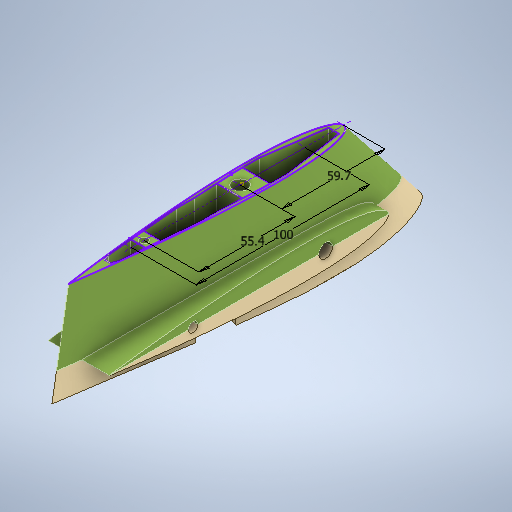
# Autodesk Inventor part: adjusted emp joint
Saved by Autodesk Inventor 2025.2 (Build 292293000, 293)
## iProperties
Created: 2025-01-22
Part Number: adjusted emp joint
Material: Generic
Document SubType Name: Modeling
Designer: User
Density: 1 g/cm^3
Appearance: Default
Author: User
Autodesk Inventor part; units mm, degrees
sketch "Sketch2" plane through (0, 0, 0) normal (0, 1, 0) x (-1, 0, 0)
  spline S0 degree 4 poles (0, 110.7513) (-0.0049, 110.7185) (-0.0278, 110.5585) (-0.067, 110.2903) (-0.1327, 109.8368) (-0.2012, 109.3601) (-0.2858, 108.7746) (-0.3847, 108.0848) (-0.4979, 107.2904) (-0.6258, 106.3921) (-0.7667, 105.3911) (-0.922, 104.2884) (-1.0895, 103.0852) (-1.2699, 101.7823) (-1.4624, 100.3817) (-1.6663, 98.8837) (-1.8812, 97.2908) (-2.107, 95.6041) (-2.3421, 93.8253) (-2.5871, 91.9562) (-2.8408, 89.9986) (-3.1031, 87.9548) (-3.3721, 85.826) (-3.6492, 83.6152) (-3.9321, 81.3238) (-4.2206, 78.9546) (-4.5149, 76.51) (-4.8135, 73.9919) (-5.116, 71.4031) (-5.4221, 68.7463) (-5.7308, 66.0238) (-6.0411, 63.2385) (-6.3537, 60.3929) (-6.6665, 57.4903) (-6.9799, 54.5331) (-7.2921, 51.5242) (-7.604, 48.4671) (-7.914, 45.3643) (-8.2212, 42.2189) (-8.5257, 39.0344) (-8.8259, 35.8132) (-9.1221, 32.5597) (-9.4131, 29.2757) (-9.6978, 25.9654) (-9.9763, 22.6318) (-10.2471, 19.2778) (-10.5104, 15.9076) (-10.7638, 12.5235) (-11.0089, 9.1296) (-11.2424, 5.7289) (-11.4659, 2.325) (-11.6768, -1.079) (-11.875, -4.4797) (-12.06, -7.8736) (-12.2312, -11.2577) (-12.3866, -14.628) (-12.5273, -17.982) (-12.651, -21.3157) (-12.7583, -24.626) (-12.8475, -27.91) (-12.9186, -31.1637) (-12.971, -34.3849) (-13.0036, -37.5695) (-13.0168, -40.7149) (-13.0094, -43.818) (-12.9816, -46.8752) (-12.9328, -49.8841) (-12.8624, -52.8415) (-12.7706, -55.7442) (-12.6573, -58.5901) (-12.5219, -61.3755) (-12.3652, -64.0983) (-12.1863, -66.7553) (-11.9859, -69.3443) (-11.7639, -71.8627) (-11.5213, -74.3077) (-11.2571, -76.6772) (-10.9725, -78.9689) (-10.6682, -81.1803) (-10.3438, -83.3094) (-10.0001, -85.3538) (-9.6381, -87.312) (-9.2577, -89.1818) (-8.8603, -90.9614) (-8.4459, -92.649) (-8.0154, -94.243) (-7.5694, -95.7422) (-7.1089, -97.1444) (-6.6339, -98.4491) (-6.1459, -99.6547) (-5.6448, -100.7602) (-5.1315, -101.7646) (-4.607, -102.6674) (-4.0703, -103.4669) (-3.5231, -104.1642) (-2.9644, -104.757) (-2.3942, -105.2456) (-1.8122, -105.6289) (-1.218, -105.9043) (-0.6135, -106.0703) (0, -106.1253) (0.6135, -106.0703) (1.218, -105.9043) (1.8122, -105.6289) (2.3942, -105.2456) (2.9644, -104.757) (3.5231, -104.1642) (4.0703, -103.4669) (4.607, -102.6674) (5.1315, -101.7646) (5.6448, -100.7602) (6.1459, -99.6547) (6.6339, -98.4491) (7.1089, -97.1444) (7.5694, -95.7422) (8.0154, -94.243) (8.4459, -92.649) (8.8603, -90.9614) (9.2577, -89.1818) (9.6381, -87.312) (10.0001, -85.3538) (10.3438, -83.3094) (10.6682, -81.1803) (10.9725, -78.9689) (11.2571, -76.6772) (11.5213, -74.3077) (11.7639, -71.8627) (11.9859, -69.3443) (12.1863, -66.7553) (12.3652, -64.0983) (12.5219, -61.3755) (12.6573, -58.5901) (12.7706, -55.7442) (12.8624, -52.8415) (12.9328, -49.8841) (12.9816, -46.8752) (13.0094, -43.818) (13.0168, -40.7149) (13.0036, -37.5695) (12.971, -34.3849) (12.9186, -31.1637) (12.8475, -27.91) (12.7583, -24.626) (12.651, -21.3157) (12.5273, -17.982) (12.3866, -14.628) (12.2312, -11.2577) (12.06, -7.8736) (11.875, -4.4797) (11.6768, -1.079) (11.4659, 2.325) (11.2424, 5.7289) (11.0089, 9.1296) (10.7638, 12.5235) (10.5104, 15.9076) (10.2471, 19.2778) (9.9763, 22.6318) (9.6978, 25.9654) (9.4131, 29.2757) (9.1221, 32.5597) (8.8259, 35.8132) (8.5257, 39.0344) (8.2212, 42.2189) (7.914, 45.3643) (7.604, 48.4671) (7.2921, 51.5242) (6.9799, 54.5331) (6.6665, 57.4903) (6.3537, 60.3929) (6.0411, 63.2385) (5.7308, 66.0238) (5.4221, 68.7463) (5.116, 71.4031) (4.8135, 73.9919) (4.5149, 76.51) (4.2206, 78.9546) (3.9321, 81.3238) (3.6492, 83.6152) (3.3721, 85.826) (3.1031, 87.9548) (2.8408, 89.9986) (2.5871, 91.9562) (2.3421, 93.8253) (2.107, 95.6041) (1.8812, 97.2908) (1.6663, 98.8837) (1.4624, 100.3817) (1.2699, 101.7823) (1.0895, 103.0852) (0.922, 104.2884) (0.7667, 105.3911) (0.6258, 106.3921) (0.4979, 107.2904) (0.3847, 108.0848) (0.2858, 108.7746) (0.2012, 109.3601) (0.1327, 109.8368) (0.067, 110.2903) (0.0278, 110.5585) (0.0049, 110.7185) (0, 110.7513) knots 0 0 0 0 0 0.003305 0.005251 0.007517 0.010057 0.012844 0.015853 0.019069 0.022477 0.026064 0.029821 0.033738 0.037807 0.04202 0.046371 0.050853 0.05546 0.060186 0.065027 0.069976 0.07503 0.080184 0.085434 0.090774 0.096201 0.101711 0.1073 0.112964 0.118699 0.124501 0.130368 0.136295 0.142278 0.148315 0.154402 0.160535 0.166711 0.172927 0.179179 0.185465 0.19178 0.198121 0.204486 0.210871 0.217273 0.223689 0.230115 0.236548 0.242985 0.249423 0.255859 0.262289 0.268711 0.275121 0.281516 0.287892 0.294248 0.300579 0.306882 0.313155 0.319394 0.325595 0.331757 0.337875 0.343946 0.349967 0.355935 0.361846 0.367698 0.373486 0.379209 0.384861 0.390441 0.395943 0.401366 0.406705 0.411957 0.417118 0.422185 0.427153 0.432019 0.436778 0.441428 0.445964 0.450381 0.454676 0.458845 0.462884 0.466789 0.470556 0.474184 0.477671 0.481017 0.484224 0.487301 0.490258 0.493116 0.495899 0.498638 0.501362 0.504101 0.506884 0.509742 0.512699 0.515776 0.518983 0.522329 0.525816 0.529444 0.533211 0.537116 0.541155 0.545324 0.549619 0.554036 0.558572 0.563222 0.567981 0.572847 0.577815 0.582882 0.588043 0.593295 0.598634 0.604057 0.609559 0.615139 0.620791 0.626514 0.632302 0.638154 0.644065 0.650033 0.656054 0.662125 0.668243 0.674405 0.680606 0.686845 0.693118 0.699421 0.705752 0.712108 0.718484 0.724879 0.731289 0.737711 0.744141 0.750577 0.757015 0.763452 0.769885 0.776311 0.782727 0.789129 0.795514 0.801879 0.80822 0.814535 0.820821 0.827073 0.833289 0.839465 0.845598 0.851685 0.857722 0.863705 0.869632 0.875499 0.881301 0.887036 0.8927 0.898289 0.903799 0.909226 0.914566 0.919816 0.92497 0.930024 0.934973 0.939814 0.94454 0.949147 0.953629 0.95798 0.962193 0.966262 0.970179 0.973936 0.977523 0.980931 0.984147 0.987156 0.989943 0.992483 0.994749 0.996695 1 1 1 1 1
  line L0 (-10.6258, 14.3547) -> (0, 14.3547)
  line L1 (0, 14.3547) -> (0, 35.8301)
  line L2 (0, 35.8301) -> (-8.8229, 35.8301)
  point P0 (0, 0)
  point P1 (0, 0)
  point P2 (0, 109.384)
  point P3 (0, -106.1025)
  point P4 (0, 0)
  point P5 (0, -106.1025)
  point P6 (-0.031, 110.5373)
  point P7 (-0.0698, 110.2701)
  point P8 (-0.124, 109.8962)
  point P9 (-0.1932, 109.4163)
  point P10 (-0.2776, 108.8308)
  point P11 (-0.3767, 108.1399)
  point P12 (-0.4901, 107.345)
  point P13 (-0.6178, 106.4461)
  point P14 (-0.7592, 105.4445)
  point P15 (-0.9143, 104.3411)
  point P16 (-1.0821, 103.1371)
  point P17 (-1.2625, 101.8336)
  point P18 (-1.4551, 100.4321)
  point P19 (-1.6591, 98.9334)
  point P20 (-1.8743, 97.3395)
  point P21 (-2.1, 95.652)
  point P22 (-2.3355, 93.8723)
  point P23 (-2.5806, 92.0021)
  point P24 (-2.8345, 90.0435)
  point P25 (-3.0967, 87.9986)
  point P26 (-3.3662, 85.8688)
  point P27 (-3.6431, 83.6567)
  point P28 (-3.9264, 81.3641)
  point P29 (-4.2152, 78.9937)
  point P30 (-4.5095, 76.5478)
  point P31 (-4.8083, 74.0284)
  point P32 (-5.111, 71.4383)
  point P33 (-5.4172, 68.7801)
  point P34 (-5.726, 66.0562)
  point P35 (-6.0368, 63.2694)
  point P36 (-6.3493, 60.4224)
  point P37 (-6.6624, 57.5183)
  point P38 (-6.9758, 54.5595)
  point P39 (-7.2885, 51.5491)
  point P40 (-7.6003, 48.4904)
  point P41 (-7.9104, 45.3859)
  point P42 (-8.2179, 42.239)
  point P43 (-8.5224, 39.0527)
  point P44 (-9.1191, 32.5746)
  point P45 (-9.4102, 29.2891)
  point P46 (-9.6951, 25.9771)
  point P47 (-9.9735, 22.6417)
  point P48 (-10.2446, 19.2861)
  point P49 (-10.5076, 15.914)
  point P50 (-10.7616, 12.5282)
  point P51 (-11.0062, 9.1325)
  point P52 (-11.2402, 5.7301)
  point P53 (-11.4633, 2.3244)
  point P54 (-11.6743, -1.0813)
  point P55 (-11.8725, -4.4837)
  point P56 (-12.0575, -7.8794)
  point P57 (-12.2284, -11.2652)
  point P58 (-12.3841, -14.6372)
  point P59 (-12.5244, -17.9928)
  point P60 (-12.6482, -21.3283)
  point P61 (-12.7551, -24.6403)
  point P62 (-12.8442, -27.9258)
  point P63 (-12.9152, -31.1812)
  point P64 (-12.9672, -34.4039)
  point P65 (-12.9997, -37.5901)
  point P66 (-13.0125, -40.7371)
  point P67 (-13.0049, -43.8416)
  point P68 (-12.9767, -46.9003)
  point P69 (-12.9275, -49.9107)
  point P70 (-12.8568, -52.8694)
  point P71 (-12.7647, -55.7735)
  point P72 (-12.6508, -58.6206)
  point P73 (-12.5151, -61.4074)
  point P74 (-12.3576, -64.1313)
  point P75 (-12.1783, -66.7895)
  point P76 (-11.9773, -69.3796)
  point P77 (-11.7548, -71.899)
  point P78 (-11.5112, -74.3449)
  point P79 (-11.2465, -76.7153)
  point P80 (-10.9611, -79.0079)
  point P81 (-10.6558, -81.22)
  point P82 (-10.3305, -83.3497)
  point P83 (-9.9859, -85.3947)
  point P84 (-9.6227, -87.3533)
  point P85 (-9.2412, -89.2234)
  point P86 (-8.8424, -91.0032)
  point P87 (-8.4267, -92.6907)
  point P88 (-7.9947, -94.2846)
  point P89 (-7.5472, -95.7833)
  point P90 (-7.0848, -97.1848)
  point P91 (-6.6082, -98.4883)
  point P92 (-6.1181, -99.6923)
  point P93 (-5.615, -100.7956)
  point P94 (-5.0998, -101.7973)
  point P95 (-4.573, -102.6961)
  point P96 (-4.035, -103.4911)
  point P97 (-3.4866, -104.182)
  point P98 (-2.9282, -104.7675)
  point P99 (-2.3602, -105.2474)
  point P100 (-1.7832, -105.6213)
  point P101 (-1.1973, -105.8884)
  point P102 (-0.6026, -106.0489)
  point P103 (0, -106.1025)
  point P104 (0.6026, -106.0489)
  point P105 (1.1973, -105.8884)
  point P106 (1.7832, -105.6213)
  point P107 (2.3602, -105.2474)
  point P108 (2.9282, -104.7675)
  point P109 (3.4866, -104.182)
  point P110 (4.035, -103.4911)
  point P111 (4.573, -102.6961)
  point P112 (5.0998, -101.7973)
  point P113 (5.615, -100.7956)
  point P114 (6.1181, -99.6923)
  point P115 (6.6082, -98.4883)
  point P116 (7.0848, -97.1848)
  point P117 (7.5472, -95.7833)
  point P118 (7.9947, -94.2846)
  point P119 (8.4267, -92.6907)
  point P120 (8.8424, -91.0032)
  point P121 (9.2412, -89.2234)
  point P122 (9.6227, -87.3533)
  point P123 (9.9859, -85.3947)
  point P124 (10.3305, -83.3497)
  point P125 (10.6558, -81.22)
  point P126 (10.9611, -79.0079)
  point P127 (11.2465, -76.7153)
  point P128 (11.5112, -74.3449)
  point P129 (11.7548, -71.899)
  point P130 (11.9773, -69.3796)
  point P131 (12.1783, -66.7895)
  point P132 (12.3576, -64.1313)
  point P133 (12.5151, -61.4074)
  point P134 (12.6508, -58.6206)
  point P135 (12.7647, -55.7735)
  point P136 (12.8568, -52.8694)
  point P137 (12.9275, -49.9107)
  point P138 (12.9767, -46.9003)
  point P139 (13.0049, -43.8416)
  point P140 (13.0125, -40.7371)
  point P141 (12.9997, -37.5901)
  point P142 (12.9672, -34.4039)
  point P143 (12.9152, -31.1812)
  point P144 (12.8442, -27.9258)
  point P145 (12.7551, -24.6403)
  point P146 (12.6482, -21.3283)
  point P147 (12.5244, -17.9928)
  point P148 (12.3841, -14.6372)
  point P149 (12.2284, -11.2652)
  point P150 (12.0575, -7.8794)
  point P151 (11.8725, -4.4837)
  point P152 (11.6743, -1.0813)
  point P153 (11.4633, 2.3244)
  point P154 (11.2402, 5.7301)
  point P155 (11.0062, 9.1325)
  point P156 (10.7616, 12.5282)
  point P157 (10.5076, 15.914)
  point P158 (10.2446, 19.2861)
  point P159 (9.9735, 22.6417)
  point P160 (9.6951, 25.9771)
  point P161 (9.4102, 29.2891)
  point P162 (9.1191, 32.5746)
  point P163 (8.8229, 35.8301)
  point P164 (8.5224, 39.0527)
  point P165 (8.2179, 42.239)
  point P166 (7.9104, 45.3859)
  point P167 (7.6003, 48.4904)
  point P168 (7.2885, 51.5491)
  point P169 (6.9758, 54.5595)
  point P170 (6.6624, 57.5183)
  point P171 (6.3493, 60.4224)
  point P172 (6.0368, 63.2694)
  point P173 (5.726, 66.0562)
  point P174 (5.4172, 68.7801)
  point P175 (5.111, 71.4383)
  point P176 (4.8083, 74.0284)
  point P177 (4.5095, 76.5478)
  point P178 (4.2152, 78.9937)
  point P179 (3.9264, 81.3641)
  point P180 (3.6431, 83.6567)
  point P181 (3.3662, 85.8688)
  point P182 (3.0967, 87.9986)
  point P183 (2.8345, 90.0435)
  point P184 (2.5806, 92.0021)
  point P185 (2.3355, 93.8723)
  point P186 (2.1, 95.652)
  point P187 (1.8743, 97.3395)
  point P188 (1.6591, 98.9334)
  point P189 (1.4551, 100.4321)
  point P190 (1.2625, 101.8336)
  point P191 (1.0821, 103.1371)
  point P192 (0.9143, 104.3411)
  point P193 (0.7592, 105.4445)
  point P194 (0.6178, 106.4461)
  point P195 (0.4901, 107.345)
  point P196 (0.3767, 108.1399)
  point P197 (0.2776, 108.8308)
  point P198 (0.1932, 109.4163)
  point P199 (0.124, 109.8962)
  constraints: 6 end point, 2 coincident, 1 horizontal, 1 parallel, 1 perpendicular, 203 other
ref_plane "Work Plane1" through (0, 60, 0) normal (0, 1, 0) x (-1, 0, 0)
sketch "Sketch3" plane through (0, 60, 0) normal (0, 1, 0) x (-1, 0, 0)
  line L0 (-3, -52.6917) -> (-8, -17.6917)
  line L1 (8, -17.6917) -> (3, -52.6917)
  line L2 (3, -52.6917) -> (-3, -52.6917)
  line L3 (-1.6981, 77.7583) -> (1.6981, 77.7583)
  line L4 (1.6981, 77.7583) -> (3, 74.3083)
  line L5 (3, 74.3083) -> (6.7391, 31.3083)
  line L6 (-6.7391, 31.3083) -> (-3, 74.3083)
  line L7 (-3, 74.3083) -> (-1.6981, 77.7583)
  spline S0 degree 4 poles (0, 100.3083) (0.0036, 100.2843) (0.0203, 100.1673) (0.049, 99.9711) (0.0971, 99.6395) (0.1472, 99.2908) (0.209, 98.8626) (0.2814, 98.358) (0.3641, 97.777) (0.4577, 97.1201) (0.5608, 96.388) (0.6743, 95.5815) (0.7968, 94.7015) (0.9287, 93.7486) (1.0695, 92.7242) (1.2187, 91.6287) (1.3758, 90.4637) (1.541, 89.2301) (1.713, 87.9291) (1.8922, 86.5621) (2.0777, 85.1304) (2.2695, 83.6356) (2.4662, 82.0787) (2.6689, 80.4618) (2.8758, 78.7859) (3.0868, 77.0532) (3.3021, 75.2653) (3.5205, 73.4236) (3.7417, 71.5303) (3.9656, 69.5872) (4.1913, 67.596) (4.4183, 65.5589) (4.6469, 63.4777) (4.8756, 61.3549) (5.1049, 59.192) (5.3332, 56.9915) (5.5613, 54.7556) (5.788, 52.4862) (6.0127, 50.1858) (6.2354, 47.8568) (6.455, 45.5009) (6.6716, 43.1214) (6.8844, 40.7196) (7.0927, 38.2986) (7.2964, 35.8604) (7.4944, 33.4075) (7.687, 30.9426) (7.8723, 28.4676) (8.0516, 25.9854) (8.2223, 23.4982) (8.3858, 21.0087) (8.54, 18.5191) (8.685, 16.0319) (8.8203, 13.5498) (8.9455, 11.0747) (9.0592, 8.6098) (9.1621, 6.1568) (9.2526, 3.7186) (9.331, 1.2976) (9.3962, -1.1042) (9.4483, -3.4839) (9.4866, -5.8398) (9.5104, -8.1689) (9.5201, -10.4694) (9.5147, -12.7388) (9.4943, -14.9748) (9.4586, -17.1754) (9.4071, -19.3384) (9.34, -21.4613) (9.2572, -23.5427) (9.1581, -25.5799) (9.0435, -27.5712) (8.9126, -29.5145) (8.7661, -31.408) (8.6037, -33.2499) (8.4263, -35.038) (8.2331, -36.771) (8.0249, -38.4471) (7.8024, -40.0644) (7.5651, -41.6216) (7.3138, -43.1168) (7.049, -44.549) (6.7708, -45.9165) (6.4801, -47.218) (6.177, -48.4523) (5.8622, -49.6181) (5.536, -50.7146) (5.1992, -51.7401) (4.8518, -52.6943) (4.4949, -53.576) (4.1284, -54.3845) (3.753, -55.1191) (3.3694, -55.7794) (2.9769, -56.3642) (2.5767, -56.8741) (2.1681, -57.3077) (1.751, -57.6651) (1.3254, -57.9454) (0.8908, -58.1468) (0.4487, -58.2682) (0, -58.3084) (-0.4487, -58.2682) (-0.8908, -58.1468) (-1.3254, -57.9454) (-1.751, -57.6651) (-2.1681, -57.3077) (-2.5767, -56.8741) (-2.9769, -56.3642) (-3.3694, -55.7794) (-3.753, -55.1191) (-4.1284, -54.3845) (-4.4949, -53.576) (-4.8518, -52.6943) (-5.1992, -51.7401) (-5.536, -50.7146) (-5.8622, -49.6181) (-6.177, -48.4523) (-6.4801, -47.218) (-6.7708, -45.9165) (-7.049, -44.549) (-7.3138, -43.1168) (-7.5651, -41.6216) (-7.8024, -40.0644) (-8.0249, -38.4471) (-8.2331, -36.771) (-8.4263, -35.038) (-8.6037, -33.2499) (-8.7661, -31.408) (-8.9126, -29.5145) (-9.0435, -27.5712) (-9.1581, -25.5799) (-9.2572, -23.5427) (-9.34, -21.4613) (-9.4071, -19.3384) (-9.4586, -17.1754) (-9.4943, -14.9748) (-9.5147, -12.7388) (-9.5201, -10.4694) (-9.5104, -8.1689) (-9.4866, -5.8398) (-9.4483, -3.4839) (-9.3962, -1.1042) (-9.331, 1.2976) (-9.2526, 3.7186) (-9.1621, 6.1568) (-9.0592, 8.6098) (-8.9455, 11.0747) (-8.8203, 13.5498) (-8.685, 16.0319) (-8.54, 18.5191) (-8.3858, 21.0087) (-8.2223, 23.4982) (-8.0516, 25.9854) (-7.8723, 28.4676) (-7.687, 30.9426) (-7.4944, 33.4075) (-7.2964, 35.8604) (-7.0927, 38.2986) (-6.8844, 40.7196) (-6.6716, 43.1214) (-6.455, 45.5009) (-6.2354, 47.8568) (-6.0127, 50.1858) (-5.788, 52.4862) (-5.5613, 54.7556) (-5.3332, 56.9915) (-5.1049, 59.192) (-4.8756, 61.3549) (-4.6469, 63.4777) (-4.4183, 65.5589) (-4.1913, 67.596) (-3.9656, 69.5872) (-3.7417, 71.5303) (-3.5205, 73.4236) (-3.3021, 75.2653) (-3.0868, 77.0532) (-2.8758, 78.7859) (-2.6689, 80.4618) (-2.4662, 82.0787) (-2.2695, 83.6356) (-2.0777, 85.1304) (-1.8922, 86.5621) (-1.713, 87.9291) (-1.541, 89.2301) (-1.3758, 90.4637) (-1.2187, 91.6287) (-1.0695, 92.7242) (-0.9287, 93.7486) (-0.7968, 94.7015) (-0.6743, 95.5815) (-0.5608, 96.388) (-0.4577, 97.1201) (-0.3641, 97.777) (-0.2814, 98.358) (-0.209, 98.8626) (-0.1472, 99.2908) (-0.0971, 99.6395) (-0.049, 99.9711) (-0.0203, 100.1673) (-0.0036, 100.2843) (0, 100.3083) knots 0 0 0 0 0 0.003305 0.005251 0.007517 0.010057 0.012844 0.015853 0.019069 0.022477 0.026064 0.029821 0.033738 0.037807 0.04202 0.046371 0.050853 0.05546 0.060186 0.065027 0.069976 0.07503 0.080184 0.085434 0.090774 0.096201 0.101711 0.1073 0.112964 0.118699 0.124501 0.130368 0.136295 0.142278 0.148315 0.154402 0.160535 0.166711 0.172927 0.179179 0.185465 0.19178 0.198121 0.204486 0.210871 0.217273 0.223689 0.230115 0.236548 0.242985 0.249423 0.255859 0.262289 0.268711 0.275121 0.281516 0.287892 0.294248 0.300579 0.306882 0.313155 0.319394 0.325595 0.331757 0.337875 0.343946 0.349967 0.355935 0.361846 0.367698 0.373486 0.379209 0.384861 0.390441 0.395943 0.401366 0.406705 0.411957 0.417118 0.422185 0.427153 0.432019 0.436778 0.441428 0.445964 0.450381 0.454676 0.458845 0.462884 0.466789 0.470556 0.474184 0.477671 0.481017 0.484224 0.487301 0.490258 0.493116 0.495899 0.498638 0.501362 0.504101 0.506884 0.509742 0.512699 0.515776 0.518983 0.522329 0.525816 0.529444 0.533211 0.537116 0.541155 0.545324 0.549619 0.554036 0.558572 0.563222 0.567981 0.572847 0.577815 0.582882 0.588043 0.593295 0.598634 0.604057 0.609559 0.615139 0.620791 0.626514 0.632302 0.638154 0.644065 0.650033 0.656054 0.662125 0.668243 0.674405 0.680606 0.686845 0.693118 0.699421 0.705752 0.712108 0.718484 0.724879 0.731289 0.737711 0.744141 0.750577 0.757015 0.763452 0.769885 0.776311 0.782727 0.789129 0.795514 0.801879 0.80822 0.814535 0.820821 0.827073 0.833289 0.839465 0.845598 0.851685 0.857722 0.863705 0.869632 0.875499 0.881301 0.887036 0.8927 0.898289 0.903799 0.909226 0.914566 0.919816 0.92497 0.930024 0.934973 0.939814 0.94454 0.949147 0.953629 0.95798 0.962193 0.966262 0.970179 0.973936 0.977523 0.980931 0.984147 0.987156 0.989943 0.992483 0.994749 0.996695 1 1 1 1 1
  line L8 (6.7391, 21.0624) -> (8, -3.4545)
  line L9 (-8, -3.4545) -> (-6.7391, 21.0624)
  line L10 (8, -3.4545) -> (8, -17.6917)
  line L11 (-8, -17.6917) -> (-8, -3.4545)
  line L12 (6.7391, 21.0624) -> (6.7391, 31.3083)
  line L13 (-6.7391, 31.3083) -> (-6.7391, 21.0624)
  line L14 (-6.5051, 34) -> (-5.8094, 42)
  line L15 (8, -8) -> (-8, -8)
  line L16 (-8, -3.4545) -> (-8, -8)
  line L17 (8, -8) -> (8, -3.4545)
  line L18 (8, -3.4545) -> (7.5652, 5)
  line L19 (-8, -3.4545) -> (-7.5138, 6)
  line L20 (8, -3.4545) -> (7.5138, 6)
  line L21 (7.5652, 5) -> (7.3175, 9.8167)
  line L22 (7.4413, 7.4083) -> (-7.4413, 7.4083)
  line L23 (-7.4413, 7.4083) -> (-7.8843, -1.2048)
  line L24 (0, 1.4083) -> (0, 56.8083) construction
  line L25 (4.9312, 52.1) -> (-4.9312, 52.1)
  line L26 (4.2355, 60.1) -> (-4.2355, 60.1)
  line L27 (0, 64) -> (0, -36) construction
  line L28 (0, -58.2917) -> (0, 1.4083) construction
  point P0 (0, 0)
  point P1 (7.8843, -1.2048)
  point P2 (5.0083, 60.1)
  dimension "d89" = 55.4
  dimension "d91" = 100
  dimension "d93" = 59.7
  constraints: 58 end point, 14 point on line, 4 vertical, 3 collinear, 3 horizontal, 2 coincident, 2 parallel, 2 perpendicular, 1 midpoint, 3 other
  measures "d89" distance of L24.start L24.end
  measures "d91" distance of L27.start L27.end
  measures "d93" distance of L28.start L24.start
ref_plane "Work Plane2" through (0, 20, 0) normal (0, 1, 0) x (-1, 0, 0)
sketch "Sketch4" plane through (0, 0, 0) normal (1, 0, 0) x (0, 1, 0)
  line L0 (20, -66.7394) -> (20.6838, -66.6456) construction
  spline S0 degree 4 poles (20, -66.7394) (20.6838, -66.6456) (21.3528, -66.3647) (22.0064, -65.8972) (22.6435, -65.2443) (23.263, -64.4074) (23.8633, -63.3886) (24.4431, -62.1901) (25.0005, -60.8149) (25.5339, -59.266) (26.0414, -57.5472) (26.5213, -55.6624) (26.9716, -53.6161) (27.3908, -51.413) (27.7773, -49.0582) (28.1295, -46.5573) (28.4463, -43.9162) (28.7266, -41.1409) (28.9696, -38.2379) (29.1748, -35.2141) (29.3419, -32.0766) (29.4708, -28.8325) (29.5619, -25.4895) (29.6156, -22.0555) (29.6156, -18.5383) (29.6156, -14.9464) (29.5617, -11.288) (29.4762, -7.5716) (29.3595, -3.806) (29.2132, 0) (29.0393, 3.8376) (28.8398, 7.6978) (28.6167, 11.5715) (28.372, 15.4498) (28.1078, 19.3235) (27.8263, 23.1837) (27.5294, 27.0213) (27.2193, 30.8273) (26.8979, 34.5929) (26.5672, 38.3093) (26.2291, 41.9677) (25.8855, 45.5597) (25.5382, 49.0768) (25.1889, 52.5108) (24.8393, 55.8538) (24.4912, 59.0978) (24.1463, 62.2354) (23.8061, 65.2592) (23.4724, 68.1622) (23.1466, 70.9375) (22.8305, 73.5786) (22.5255, 76.0795) (22.2332, 78.4343) (21.9552, 80.6374) (21.693, 82.6837) (21.448, 84.5685) (21.2215, 86.2873) (21.015, 87.8362) (20.8295, 89.2114) (20.6664, 90.4099) (20.5265, 91.4287) (20.4108, 92.2656) (20.32, 92.9185) (20.2547, 93.386) (20.2154, 93.6669) (20.2022, 93.7606) (20, 94.7236) (19.7978, 93.7606) (19.7846, 93.6669) (19.7453, 93.386) (19.68, 92.9185) (19.5892, 92.2656) (19.4735, 91.4287) (19.3336, 90.4099) (19.1704, 89.2114) (18.985, 87.8362) (18.7785, 86.2873) (18.552, 84.5685) (18.307, 82.6837) (18.0447, 80.6374) (17.7667, 78.4343) (17.4745, 76.0795) (17.1695, 73.5786) (16.8534, 70.9375) (16.5276, 68.1622) (16.1939, 65.2592) (15.8537, 62.2354) (15.5087, 59.0978) (15.1607, 55.8538) (14.8111, 52.5108) (14.4618, 49.0768) (14.1145, 45.5597) (13.7708, 41.9677) (13.4327, 38.3093) (13.1021, 34.5929) (12.7807, 30.8273) (12.4705, 27.0213) (12.1737, 23.1837) (11.8922, 19.3235) (11.628, 15.4498) (11.3833, 11.5715) (11.1601, 7.6978) (10.9606, 3.8376) (10.7868, 0) (10.6405, -3.806) (10.5238, -7.5716) (10.4382, -11.288) (10.3856, -14.9464) (10.3856, -18.5384) (10.3856, -22.0555) (10.4381, -25.4895) (10.5292, -28.8325) (10.6581, -32.0766) (10.8252, -35.2141) (11.0304, -38.2379) (11.2734, -41.1409) (11.5537, -43.9162) (11.8705, -46.5573) (12.2227, -49.0582) (12.6091, -51.413) (13.0283, -53.6161) (13.4787, -55.6624) (13.9585, -57.5472) (14.4661, -59.266) (14.9995, -60.8149) (15.5569, -62.1901) (16.1367, -63.3886) (16.737, -64.4074) (17.3565, -65.2443) (17.9936, -65.8972) (18.6472, -66.3647) (19.3162, -66.6456) (20, -66.7394) knots 1 1 1 1 1 2 3 4 5 6 7 8 9 10 11 12 13 14 15 16 17 18 19 20 21 22 23 24 25 26 27 28 29 30 31 32 33 34 35 36 37 38 39 40 41 42 43 44 45 46 47 48 49 50 51 52 53 54 55 56 57 58 59 60 61 62 63 64 65 66 67 68 69 70 71 72 73 74 75 76 77 78 79 80 81 82 83 84 85 86 87 88 89 90 91 92 93 94 95 96 97 98 99 100 101 102 103 104 105 106 107 108 109 110 111 112 113 114 115 116 117 118 119 120 121 122 123 124 125 126 127 128 129 130 130 130 130 130
  line L1 (20.6838, -66.6456) -> (21.3528, -66.3647) construction
  line L2 (21.3528, -66.3647) -> (22.0064, -65.8972) construction
  line L3 (22.0064, -65.8972) -> (22.6435, -65.2443) construction
  line L4 (22.6435, -65.2443) -> (23.263, -64.4074) construction
  line L5 (23.263, -64.4074) -> (23.8633, -63.3886) construction
  line L6 (23.8633, -63.3886) -> (24.4431, -62.1901) construction
  line L7 (24.4431, -62.1901) -> (25.0005, -60.8149) construction
  line L8 (25.0005, -60.8149) -> (25.5339, -59.266) construction
  line L9 (25.5339, -59.266) -> (26.0414, -57.5472) construction
  line L10 (26.0414, -57.5472) -> (26.5213, -55.6624) construction
  line L11 (26.5213, -55.6624) -> (26.9716, -53.6161) construction
  line L12 (26.9716, -53.6161) -> (27.3908, -51.413) construction
  line L13 (27.3908, -51.413) -> (27.7773, -49.0582) construction
  line L14 (27.7773, -49.0582) -> (28.1295, -46.5573) construction
  line L15 (28.1295, -46.5573) -> (28.4463, -43.9162) construction
  line L16 (28.4463, -43.9162) -> (28.7266, -41.1409) construction
  line L17 (28.7266, -41.1409) -> (28.9696, -38.2379) construction
  line L18 (28.9696, -38.2379) -> (29.1748, -35.2141) construction
  line L19 (29.1748, -35.2141) -> (29.3419, -32.0766) construction
  line L20 (29.3419, -32.0766) -> (29.4708, -28.8325) construction
  line L21 (29.4708, -28.8325) -> (29.5619, -25.4895) construction
  line L22 (29.5619, -25.4895) -> (29.6156, -22.0555) construction
  line L23 (29.6156, -22.0555) -> (29.6156, -18.5383) construction
  line L24 (29.6156, -18.5383) -> (29.6156, -14.9464) construction
  line L25 (29.6156, -14.9464) -> (29.5617, -11.288) construction
  line L26 (29.5617, -11.288) -> (29.4762, -7.5716) construction
  line L27 (29.4762, -7.5716) -> (29.3595, -3.806) construction
  line L28 (29.3595, -3.806) -> (29.2132, 0) construction
  line L29 (29.2132, 0) -> (29.0393, 3.8376) construction
  line L30 (29.0393, 3.8376) -> (28.8398, 7.6978) construction
  line L31 (28.8398, 7.6978) -> (28.6167, 11.5715) construction
  line L32 (28.6167, 11.5715) -> (28.372, 15.4498) construction
  line L33 (28.372, 15.4498) -> (28.1078, 19.3235) construction
  line L34 (28.1078, 19.3235) -> (27.8263, 23.1837) construction
  line L35 (27.8263, 23.1837) -> (27.5294, 27.0213) construction
  line L36 (27.5294, 27.0213) -> (27.2193, 30.8273) construction
  line L37 (27.2193, 30.8273) -> (26.8979, 34.5929) construction
  line L38 (26.8979, 34.5929) -> (26.5672, 38.3093) construction
  line L39 (26.5672, 38.3093) -> (26.2291, 41.9677) construction
  line L40 (26.2291, 41.9677) -> (25.8855, 45.5597) construction
  line L41 (25.8855, 45.5597) -> (25.5382, 49.0768) construction
  line L42 (25.5382, 49.0768) -> (25.1889, 52.5108) construction
  line L43 (25.1889, 52.5108) -> (24.8393, 55.8538) construction
  line L44 (24.8393, 55.8538) -> (24.4912, 59.0978) construction
  line L45 (24.4912, 59.0978) -> (24.1463, 62.2354) construction
  line L46 (24.1463, 62.2354) -> (23.8061, 65.2592) construction
  line L47 (23.8061, 65.2592) -> (23.4724, 68.1622) construction
  line L48 (23.4724, 68.1622) -> (23.1466, 70.9375) construction
  line L49 (23.1466, 70.9375) -> (22.8305, 73.5786) construction
  line L50 (22.8305, 73.5786) -> (22.5255, 76.0795) construction
  line L51 (22.5255, 76.0795) -> (22.2332, 78.4343) construction
  line L52 (22.2332, 78.4343) -> (21.9552, 80.6374) construction
  line L53 (21.9552, 80.6374) -> (21.693, 82.6837) construction
  line L54 (21.693, 82.6837) -> (21.448, 84.5685) construction
  line L55 (21.448, 84.5685) -> (21.2215, 86.2873) construction
  line L56 (21.2215, 86.2873) -> (21.015, 87.8362) construction
  line L57 (21.015, 87.8362) -> (20.8295, 89.2114) construction
  line L58 (20.8295, 89.2114) -> (20.6664, 90.4099) construction
  line L59 (20.6664, 90.4099) -> (20.5265, 91.4287) construction
  line L60 (20.5265, 91.4287) -> (20.4108, 92.2656) construction
  line L61 (20.4108, 92.2656) -> (20.32, 92.9185) construction
  line L62 (20.32, 92.9185) -> (20.2547, 93.386) construction
  line L63 (20.2547, 93.386) -> (20.2154, 93.6669) construction
  line L64 (20.2154, 93.6669) -> (20.2022, 93.7606) construction
  line L65 (20.2022, 93.7606) -> (20, 94.7236) construction
  line L66 (20, 94.7236) -> (19.7978, 93.7606) construction
  line L67 (19.7978, 93.7606) -> (19.7846, 93.6669) construction
  line L68 (19.7846, 93.6669) -> (19.7453, 93.386) construction
  line L69 (19.7453, 93.386) -> (19.68, 92.9185) construction
  line L70 (19.68, 92.9185) -> (19.5892, 92.2656) construction
  line L71 (19.5892, 92.2656) -> (19.4735, 91.4287) construction
  line L72 (19.4735, 91.4287) -> (19.3336, 90.4099) construction
  line L73 (19.3336, 90.4099) -> (19.1704, 89.2114) construction
  line L74 (19.1704, 89.2114) -> (18.985, 87.8362) construction
  line L75 (18.985, 87.8362) -> (18.7785, 86.2873) construction
  line L76 (18.7785, 86.2873) -> (18.552, 84.5685) construction
  line L77 (18.552, 84.5685) -> (18.307, 82.6837) construction
  line L78 (18.307, 82.6837) -> (18.0447, 80.6374) construction
  line L79 (18.0447, 80.6374) -> (17.7667, 78.4343) construction
  line L80 (17.7667, 78.4343) -> (17.4745, 76.0795) construction
  line L81 (17.4745, 76.0795) -> (17.1695, 73.5786) construction
  line L82 (17.1695, 73.5786) -> (16.8534, 70.9375) construction
  line L83 (16.8534, 70.9375) -> (16.5276, 68.1622) construction
  line L84 (16.5276, 68.1622) -> (16.1939, 65.2592) construction
  line L85 (16.1939, 65.2592) -> (15.8537, 62.2354) construction
  line L86 (15.8537, 62.2354) -> (15.5087, 59.0978) construction
  line L87 (15.5087, 59.0978) -> (15.1607, 55.8538) construction
  line L88 (15.1607, 55.8538) -> (14.8111, 52.5108) construction
  line L89 (14.8111, 52.5108) -> (14.4618, 49.0768) construction
  line L90 (14.4618, 49.0768) -> (14.1145, 45.5597) construction
  line L91 (14.1145, 45.5597) -> (13.7708, 41.9677) construction
  line L92 (13.7708, 41.9677) -> (13.4327, 38.3093) construction
  line L93 (13.4327, 38.3093) -> (13.1021, 34.5929) construction
  line L94 (13.1021, 34.5929) -> (12.7807, 30.8273) construction
  line L95 (12.7807, 30.8273) -> (12.4705, 27.0213) construction
  line L96 (12.4705, 27.0213) -> (12.1737, 23.1837) construction
  line L97 (12.1737, 23.1837) -> (11.8922, 19.3235) construction
  line L98 (11.8922, 19.3235) -> (11.628, 15.4498) construction
  line L99 (11.628, 15.4498) -> (11.3833, 11.5715) construction
  line L100 (11.3833, 11.5715) -> (11.1601, 7.6978) construction
  line L101 (11.1601, 7.6978) -> (10.9606, 3.8376) construction
  line L102 (10.9606, 3.8376) -> (10.7868, 0) construction
  line L103 (10.7868, 0) -> (10.6405, -3.806) construction
  line L104 (10.6405, -3.806) -> (10.5238, -7.5716) construction
  line L105 (10.5238, -7.5716) -> (10.4382, -11.288) construction
  line L106 (10.4382, -11.288) -> (10.3856, -14.9464) construction
  line L107 (10.3856, -14.9464) -> (10.3856, -18.5384) construction
  line L108 (10.3856, -18.5384) -> (10.3856, -22.0555) construction
  line L109 (10.3856, -22.0555) -> (10.4381, -25.4895) construction
  line L110 (10.4381, -25.4895) -> (10.5292, -28.8325) construction
  line L111 (10.5292, -28.8325) -> (10.6581, -32.0766) construction
  line L112 (10.6581, -32.0766) -> (10.8252, -35.2141) construction
  line L113 (10.8252, -35.2141) -> (11.0304, -38.2379) construction
  line L114 (11.0304, -38.2379) -> (11.2734, -41.1409) construction
  line L115 (11.2734, -41.1409) -> (11.5537, -43.9162) construction
  line L116 (11.5537, -43.9162) -> (11.8705, -46.5573) construction
  line L117 (11.8705, -46.5573) -> (12.2227, -49.0582) construction
  line L118 (12.2227, -49.0582) -> (12.6091, -51.413) construction
  line L119 (12.6091, -51.413) -> (13.0283, -53.6161) construction
  line L120 (13.0283, -53.6161) -> (13.4787, -55.6624) construction
  line L121 (13.4787, -55.6624) -> (13.9585, -57.5472) construction
  line L122 (13.9585, -57.5472) -> (14.4661, -59.266) construction
  line L123 (14.4661, -59.266) -> (14.9995, -60.8149) construction
  line L124 (14.9995, -60.8149) -> (15.5569, -62.1901) construction
  line L125 (15.5569, -62.1901) -> (16.1367, -63.3886) construction
  line L126 (16.1367, -63.3886) -> (16.737, -64.4074) construction
  line L127 (16.737, -64.4074) -> (17.3565, -65.2443) construction
  line L128 (17.3565, -65.2443) -> (17.9936, -65.8972) construction
  line L129 (17.9936, -65.8972) -> (18.6472, -66.3647) construction
  line L130 (18.6472, -66.3647) -> (19.3162, -66.6456) construction
  line L131 (19.3162, -66.6456) -> (20, -66.7394) construction
  line L132 (20, -66.7394) -> (20, -30.4894) construction
  line L133 (20, -66.7394) -> (20, 45.9606) construction
  point P0 (20, -66.7394)
  point P1 (20, -66.7394)
  constraints: 132 coincident, 4 end point, 2 vertical, 1 other
loft "Loft1" add profiles "Sketch2", "Sketch3" contours all / L0 L11 L15 L10 L1 L2 | L11 L9 L22 L8 L10 L15 | L9 L13 L6 L25 L5 L12 L8 L22 | L6 L26 L5 L25 | L6 L7 L3 L4 L5 L26 | S0
extrude "Extrusion1" add sketch "Sketch4" along normal mid plane 35
hole "Hole1" at (0, 20, -30.4894) direction (-1, 0, 0) diameter 8 end through all both
hole "Hole2" at (0, 20, 45.9606) direction (-1, 0, 0) diameter 5.5 end through all both
hole "Hole5" at (0, 60, 64) at (0, 60, -36) direction (0, -1, 0) diameter 5.5 end through all
extrude "Extrusion3" cut sketch "Sketch2" along normal blind 12.75 contours L2 L1 L0 S0 picked at (-6.4829, 21.5132)
ref_plane "Work Plane3" through (0, 0, -127.5) normal (0, 0, 1) x (1, 0, 0)
sketch "Sketch5" plane through (0, 0, -127.5) normal (0, 0, 1) x (1, 0, 0)
  circle A0 centre (0, -13.4363) radius 18.75
  point P0 (0, 0)
  dimension "d63" = 37.5
  constraints: 1 centre point
  measures "d63" diameter of A0
extrude "Extrusion4" cut sketch "Sketch5" along normal blind 367 draft -0.124
sketch "Sketch1" plane through (0, 0, 0) normal (0, 1, 0) x (-1, 0, 0)
  point P0 (0, 0)
split body "Split1" result two bodies by plane through (0, 20, 0) normal (0, 1, 0) first body at (6.5752, 48.4932, 41.7932)
extrude "Extrusion5" cut sketch "Sketch3" against normal blind 30 contours L0 L11 L15 L10 L1 L2 | L9 L13 L6 L25 L5 L12 L8 L22 | L6 L7 L3 L4 L5 L26 bodies 2
hole "Hole7" at (0, 60, 56.8083) direction (0, -1, 0) diameter 4.5 depth 35 tip angle 118 bodies 2
hole "Hole8" at (0, 60, 1.4083) direction (0, -1, 0) diameter 8.5 depth 35 bodies 2
sketch "Sketch6" plane through (0, 12.75, 0) normal (0, -1, 0) x (1, 0, 0)
  line L0 (0, 35.8301) -> (8.5073, 35.8301) projected
  line L1 (-5.7464, 35.8301) -> (-5.7464, 14.8301)
  line L2 (-5.7464, 14.8301) -> (4.2536, 14.8301)
  line L3 (4.2536, 14.8301) -> (4.2536, 34)
  line L4 (6.5051, 34) -> (-6.5051, 34) projected
  line L5 (4.2536, 34) -> (-5.7464, 34)
  line L6 (4.2536, 34) -> (-5.7464, 34)
  point P0 (0, 0)
  dimension "d85" = 10
  dimension "d86" = 21
  constraints: 10 end point, 1 collinear, 1 parallel, 1 point on line
  measures "d85" distance of L2.end L1.end
  measures "d86" distance of L1.end L1.start
extrude "Extrusion6" cut sketch "Sketch6" along normal mid plane 69.75 bodies 3 2
sketch "Sketch7" plane through (0, 60, 21.0083) normal (0, 1, 0) x (0.9890787, 0, 0.1473884)
  point P0 (-3.0964, 20.7788)
body "Solid2"
body "Solid3"
